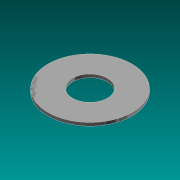
# Autodesk Inventor part: UW-0308-03
Saved by Autodesk Inventor 2016 (Build 200138000, 138)
## iProperties
Created: 2016-05-27
Part Number: UW-0308-03
Material: ステンレス鋼 AISI 302
Document SubType Name: Modeling
Designer: hiroaki
Density: 8 g/cm^3
Appearance: 半つや出し
Mass: 0.10011 g
Surface Area: 0.94075 cm^2
Volume: 0.0125137 cm^3
Author: hiroaki
Autodesk Inventor part; units mm, degrees
ref_plane "YZ Plane" through (0, 0, 0) normal (1, 0, 0) x (0, 1, 0)
ref_plane "XZ Plane" through (0, 0, 0) normal (0, 1, 0) x (-1, 0, 0)
ref_plane "XY Plane" through (0, 0, 0) normal (0, 0, 1) x (1, 0, 0)
sketch "スケッチ1" plane through (0, 0, 0) normal (0, 0, 1) x (1, 0, 0)
  circle A0 centre (0, 0) radius 4
  circle A1 centre (0, 0) radius 1.65
  dimension "d0" = 8
  dimension "d1" = 3.3
  constraints: 2 centre point, 2 coincident
  measures "d0" diameter of A0
  measures "d1" diameter of A1
extrude "押し出し1" add sketch "スケッチ1" along normal blind 0.3
